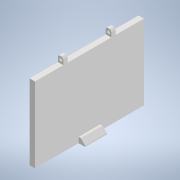
# Autodesk Inventor part: box_door
Saved by Autodesk Inventor 2020 (Build 240168000, 168)
## iProperties
Created: 2020-03-03
Part Number: box_door
Material: Generic
Document SubType Name: Modeling
Designer: Luka
Density: 1 g/cm^3
Appearance: Default
Author: Luka
Autodesk Inventor part; units mm, degrees
ref_plane "YZ Plane" through (0, 0, 0) normal (1, 0, 0) x (0, 1, 0)
ref_plane "XZ Plane" through (0, 0, 0) normal (0, 1, 0) x (-1, 0, 0)
ref_plane "XY Plane" through (0, 0, 0) normal (0, 0, 1) x (1, 0, 0)
sketch "Sketch1" plane through (0, 0, 0) normal (0, 1, 0) x (-1, 0, 0)
  line L0 (42.3333, 428.0371) -> (37.3333, 428.0371)
  line L1 (37.3333, 428.0371) -> (37.3333, 330.0371)
  line L2 (37.3333, 330.0371) -> (42.3333, 330.0371)
  line L3 (42.3333, 330.0371) -> (42.3333, 428.0371)
  point P0 (0, 0)
  dimension "d0" = 5
  dimension "d1" = 98
  constraints: 8 end point, 2 parallel, 1 horizontal, 1 perpendicular
  measures "d0" distance of L0.start L0.end
  measures "d1" distance of L2.end L0.start
extrude "Extrusion1" add sketch "Sketch1" along normal blind 68
move or copy body "Move Body1" bodies to move or copy 1 copy no translate (15.875, -14.288, -387.35)
sketch "Sketch2" plane through (0, 68, 0) normal (0, 1, 0) x (1, 0, 0)
  line L0 (-26.4583, 57.3129) -> (-26.4583, -40.6871) projected
  line L1 (-21.4583, -40.6871) -> (-21.4583, 57.3129) projected
  line L2 (-26.4583, -15.6871) -> (-21.4583, -15.6871)
  line L3 (-21.4583, -15.6871) -> (-21.4583, -11.6871)
  line L4 (-21.4583, -11.6871) -> (-26.4583, -11.6871)
  line L5 (-26.4583, -11.6871) -> (-26.4583, -15.6871)
  line L6 (-26.4583, 28.3129) -> (-21.4583, 28.3129)
  line L7 (-21.4583, 28.3129) -> (-21.4583, 32.3129)
  line L8 (-21.4583, 32.3129) -> (-26.4583, 32.3129)
  line L9 (-26.4583, 32.3129) -> (-26.4583, 28.3129)
  line L10 (-26.4583, -40.6871) -> (-21.4583, -40.6871) projected
  line L11 (-21.4583, 57.3129) -> (-26.4583, 57.3129) projected
  line L12 (-21.4583, -40.6871) -> (-22.4583, -40.6871)
  line L13 (-22.4583, -40.6871) -> (-22.4583, 57.3129)
  line L14 (-22.4583, 57.3129) -> (-21.4583, 57.3129)
  line L15 (-21.4583, 57.3129) -> (-21.4583, -40.6871)
  point P0 (0, 0)
  point P1 (-26.4583, 32.3129)
  point P2 (-26.4583, 28.3129)
  point P3 (-26.4583, -11.6871)
  dimension "d7" = 29
  dimension "d8" = 29
  dimension "d9" = 25
  dimension "d10" = 25
  dimension "d26" = 1
  constraints: 24 end point, 6 parallel, 5 point on line, 3 horizontal, 3 perpendicular
  measures "d7" distance between parallel lines of L4 L10
  measures "d8" distance between parallel lines of L11 L6
  measures "d9" distance between parallel lines of L11 L8
  measures "d10" distance between parallel lines of L10 L2
  measures "d26" distance between parallel lines of L13 L1
move or copy body "Move Body2" bodies to move or copy 1 copy no translate (0, 14.288, 0)
extrude "Extrusion2" add sketch "Sketch2" along normal blind 6 contours L8 L13 L6 L0 | L8 L1 L6 L13 | L4 L13 L2 L0 | L4 L1 L2 L13
sketch "Sketch4" plane through (-26.4583, 68, 15.6871) normal (0, 0, 1) x (1, 0, 0)
  line L0 (0, 6) -> (5, 6) projected
  line L1 (5, 0) -> (5, 6) projected
  point P0 (26.4583, -68)
  point P1 (2.5, 3)
  dimension "d17" = 3
  dimension "d18" = 2.5
  measures "d17" distance from line of L0 point (2.5, 3)
  measures "d18" distance from line of L1 point (2.5, 3)
hole "Hole1" at (-23.9583, 71, 15.6871) direction (0, 0, -1) diameter 2.5 end through all
sketch "Sketch5" plane through (-21.4583, 0, 40.6871) normal (1, 0, 0) x (0, 0, -1)
  line L0 (40, 5) -> (58, 5)
  line L1 (58, 5) -> (58, 0)
  line L2 (58, 0) -> (40, 0)
  line L3 (40, 0) -> (40, 5)
  line L4 (0, 0) -> (98, 0) projected
  line L5 (0, 0) -> (0, 68) projected
  line L6 (98, 0) -> (98, 68) projected
  point P0 (40.6871, 0)
  dimension "d27" = 0
  dimension "d28" = 5
  dimension "d29" = 40
  dimension "d30" = 40
  constraints: 8 end point, 2 parallel, 1 horizontal, 1 perpendicular
  measures "d27" distance between parallel lines of L4 L2
  measures "d28" distance between parallel lines of L4 L0
  measures "d29" distance between parallel lines of L5 L3
  measures "d30" distance between parallel lines of L6 L1
extrude "Extrusion3" add sketch "Sketch5" along normal blind 6
chamfer "Chamfer1" distance 4 angle 45 1 edges at (-15.4583, 5, -8.3129)
fillet "Fillet1" radius 2.5 4 edges at (-21.4583, 74, -30.3129) (-21.4583, 74, 13.6871) (-26.4583, 74, -30.3129) (-26.4583, 74, 13.6871)
body "Solid1"
